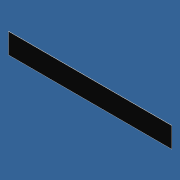
# Autodesk Inventor part: Velcro
Saved by Autodesk Inventor 2012 (Build 160160000, 160)
## iProperties
Created: 2010-10-06
Part Number: Velcro
Document SubType Name: Modeling
Designer: mcyr
Density: 1 g/cm^3
Material: Default
Author: mcyr
Autodesk Inventor part; units mm, degrees
ref_plane "YZ Plane" through (0, 0, 0) normal (1, 0, 0) x (0, 1, 0)
ref_plane "XZ Plane" through (0, 0, 0) normal (0, 1, 0) x (-1, 0, 0)
ref_plane "XY Plane" through (0, 0, 0) normal (0, 0, 1) x (1, 0, 0)
sketch "Sketch1" plane through (0, 0, 0) normal (0, 0, 1) x (1, 0, 0)
  line L0 (-25.5063, 25.0723) -> (380.8937, 25.0723)
  line L1 (380.8937, 25.0723) -> (380.8937, -25.7277)
  line L2 (380.8937, -25.7277) -> (-25.5063, -25.7277)
  line L3 (-25.5063, -25.7277) -> (-25.5063, 25.0723)
  point P0 (0, 0)
  dimension "d0" = 406.4
  dimension "d1" = 50.8
  constraints: 8 end point, 2 parallel, 1 horizontal, 1 perpendicular
  measures "d0" distance of L0.start L0.end
  measures "d1" distance of L2.end L0.start
extrude "Extrusion1" add sketch "Sketch1" along normal blind 0.635
body "Solid1"
